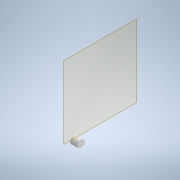
# Autodesk Inventor part: 작은 원통
Saved by Autodesk Inventor 2022 (Build 260153000, 153)
## iProperties
Created: 2022-10-28
Part Number: 작은 원통
Material: 일반
Document SubType Name: Modeling
Designer: gogin
Density: 1 g/cm^3
Appearance: 기본값
Author: gogin
Autodesk Inventor part; units mm, degrees
ref_plane "YZ Plane" through (0, 0, 0) normal (1, 0, 0) x (0, 1, 0)
ref_plane "XZ Plane" through (0, 0, 0) normal (0, 1, 0) x (-1, 0, 0)
ref_plane "XY Plane" through (0, 0, 0) normal (0, 0, 1) x (1, 0, 0)
sketch "스케치1" plane through (0, 0, 0) normal (1, 0, 0) x (0, 1, 0)
  circle A0 centre (1, -1) radius 0.5
  point P0 (0, 0)
  dimension "d0" = 1
  dimension "d1" = 1
  dimension "d2" = 1
  constraints: 1 centre point
  measures "d0" diameter of A0
  measures "d1" horizontal distance of point (0, 0) A0.centre
  measures "d2" horizontal distance of A0.centre point (0, 0)
extrude "돌출1" add sketch "스케치1" along normal blind 1
ref_plane "작업 평면2" through (2.77, 8.8098, -1.8323) normal (1, 0, 0) x (0, 1, 0)
